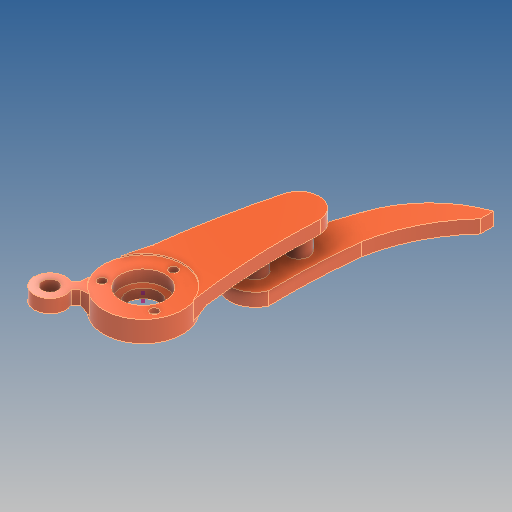
# Autodesk Inventor part: 01-03-01 Zange links nue
Saved by Autodesk Inventor 2026.2 (Build 302298000, 298)
## iProperties
Created: 2025-12-11
Part Number: 01-03-01 Zange links nue
Material: Phenolharz
Document SubType Name: Modeling
Designer: Schally
Density: 1.38 g/cm^3
Appearance: Glatt - Hellorange
Author: Schally
Autodesk Inventor part; units mm, degrees
sketch "Skizze10" plane through (0, 0, 0) normal (1, 0, 0) x (0, 1, 0)
  line L0 (-1.4, 0) -> (8.4, 0) projected
  line L1 (0, -13.2) -> (0, 2.2) projected
  line L2 (2, -2.5) -> (7, -2.5)
  line L3 (7, -2.5) -> (7, -8.5)
  line L4 (7, -8.5) -> (2, -8.5)
  line L5 (2, -8.5) -> (2, -2.5)
  point P0 (0, 0)
  point P1 (0, -11)
  dimension "d135" = 8.5
  dimension "d137" = 5
  dimension "d138" = 2
  dimension "d145" = 2.5
  constraints: 8 end point, 2 parallel, 1 horizontal, 1 perpendicular, 1 point on line
  measures "d135" distance between parallel lines of L0 L4
  measures "d137" distance between parallel lines of L5 L3
  measures "d138" distance between parallel lines of L1 L5
  measures "d145" distance between parallel lines of L0 L2
revolve "Umdrehung2" add sketch "Skizze10" angle 360 about axis through (0, -10, 0) along (0, 1, 0)
ref_plane "Arbeitsebene2" through (0, 6, 0) normal (0, 1, 0) x (1, 0, 0)
ref_plane "Arbeitsebene3" through (0, 4.5, 0) normal (0, 1, 0) x (1, 0, 0)
sketch "Skizze12" plane through (0, 4.5, 0) normal (0, 1, 0) x (1, 0, 0)
  arc A0 (3.5, 80) -> (-11.5, 15.25) centre (296.2619, -21.9337) ccw projected
  arc A1 (28, 100) -> (13, 70) centre (72.0267, 59.2367) ccw projected
  line L0 (28, 100) -> (28, 105) projected
  arc A2 (28, 105) -> (3.5, 80) centre (41.4387, 67.3251) ccw projected
  circle A3 centre (0, 0) radius 15
  arc A4 (13, 70) -> (15, 0) centre (261.1443, 42.0613) ccw
  arc A5 (-11.5, 15.25) -> (-15, 0) centre (120.624, -23.1002) ccw
  circle A6 centre (0, 0) radius 8.5 projected
  line L1 (0, 0) -> (-17.6777, -17.6777)
  line L2 (-87.6656, 0) -> (360.2498, 0) projected
  line L3 (0, 134.1222) -> (0, -49.9776) projected
  circle A7 centre (-17.6777, -17.6777) radius 6
  circle A8 centre (-17.6777, -17.6777) radius 3
  line L4 (1.4142, -1.4142) -> (-12.7279, -15.5563)
  line L5 (-1.4142, 1.4142) -> (-15.5563, -12.7279)
  point P0 (-16.4, 0)
  point P1 (-11.9261, -9.0977)
  point P2 (-15.0919, -12.2635)
  point P3 (-12.2635, -15.0919)
  point P4 (-9.0977, -11.9261)
  dimension "d147" = 30
  dimension "d148" = 45
  dimension "d149" = 25
  dimension "d150" = 12
  dimension "d152" = 3
  dimension "d153" = 2
  dimension "d154" = 2
  constraints: 6 end point, 6 point on circle, 5 centre point, 3 coincident, 2 parallel
  measures "d147" diameter of A3
  measures "d148" angle of L1 L3
  measures "d149" distance of L1.start L1.end
  measures "d150" diameter of A7
  measures "d152" radial gap between concentric circles of A7 A8
  measures "d153" distance between parallel lines of L1 L4
  measures "d154" distance between parallel lines of L1 L5
sketch "Skizze13" plane through (0, 4.5, 0) normal (0, 1, 0) x (1, 0, 0)
  point P0 (0, 0)
extrude "Extrusion8" add sketch "Skizze12" along normal mid plane 5 contours A2 L0 A1 A4 A3 L3 A0 | L3 A3 A5 A0 | L3 A6 L2 A5 A3 | A3 A4 L2 A6 L3 | L3 L2 A6 | A6 L2 L3 | L2 A6 L5 A3 | A3 L3 A6 L2 | A6 L3 L2 | L2 L5 A6 | L3 L4 A6 L1 | L1 A6 L5 L2 | L5 A6 L1 A3 | A3 L1 A7 L5 | A3 L4 A6 L3 | A6 L4 L3 | A6 L4 A3 L1 | A3 L4 A7 L1 | A7
sketch "Skizze14" plane through (0, 4.5, 0) normal (0, 1, 0) x (1, 0, 0)
  circle A0 centre (0, 0) radius 2.5
  dimension "d157" = 5
  constraints: 1 centre point, 1 coincident
  measures "d157" diameter of A0
extrude "Extrusion9" cut sketch "Skizze14" along normal mid plane 20
sketch "Skizze15" plane through (0, 4.5, 0) normal (0, 1, 0) x (1, 0, 0)
  arc A0 (-11.5, 15.25) -> (-15, 0) centre (120.624, -23.1002) ccw projected
  circle A1 centre (0, 0) radius 15
  constraints: 1 coincident, 1 horizontal alignment, 2 other
extrude "Extrusion10" add sketch "Skizze15" along normal mid plane 12
sketch "Skizze16" plane through (0, 4.5, 0) normal (0, 1, 0) x (1, 0, 0)
  circle A0 centre (0, 0) radius 6
  dimension "d162" = 12
  constraints: 1 centre point, 1 coincident
  measures "d162" diameter of A0
extrude "Extrusion11" cut sketch "Skizze16" along normal mid plane 12
sketch "Skizze17" plane through (0, 4.5, 0) normal (0, 1, 0) x (1, 0, 0)
  circle A0 centre (0, 0) radius 8.5
  dimension "d165" = 17
  constraints: 1 centre point, 1 coincident
  measures "d165" diameter of A0
extrude "Extrusion12" cut sketch "Skizze17" along normal mid plane 5
chamfer "Fasen7" distance 2 angle 45 8 edges at (-10.6066, 7, 10.6066) (-9.0977, 5.75, 11.9261) (-9.0977, 3.25, 11.9261) (-10.6066, 2, 10.6066) (0.4428, 2, -14.9935) (0.4428, 7, -14.9935) (-11.9261, 5.75, 9.0977) (-11.9261, 3.25, 9.0977)
sketch "Skizze18" plane through (28, 2, -105) normal (0, -1, 0) x (1, 0, 0)
  point P0 (-28, 105)
ref_plane "Arbeitsebene4" through (28, -7, -105) normal (0, -1, 0) x (1, 0, 0)
sketch "Skizze20" plane through (28, 2, -105) normal (0, -1, 0) x (1, 0, 0)
  circle A0 centre (-24, 50) radius 4
  circle A1 centre (-25.5, 65) radius 4
  point P0 (-28, 105)
  dimension "d188" = 8
  dimension "d189" = 8
  dimension "d192" = 1.5
  dimension "d193" = 15
  constraints: 2 centre point
  measures "d188" diameter of A0
  measures "d189" diameter of A1
  measures "d192" horizontal distance of A1.centre A0.centre
  measures "d193" vertical distance of A1.centre A0.centre
extrude "Extrusion14" add sketch "Skizze20" along normal blind 9
sketch "Skizze19" plane through (28, -7, -105) normal (0, -1, 0) x (1, 0, 0)
  arc A0 (-24.5, 25) -> (0, 0) centre (13.4387, 37.6749) ccw projected
  arc A1 (-15, 35) -> (0, 5) centre (44.0267, 45.7633) ccw projected
  line L0 (0, 0) -> (0, 5) projected
  line L1 (-15, 35) -> (-24.5, 25)
  arc A2 (-39.5, 89.75) -> (-24.5, 25) centre (268.2619, 126.9337) ccw projected
  arc A3 (-14.5526, 94.5996) -> (-15, 35) centre (233.1443, 62.9387) ccw projected
  line L2 (-27, 80) -> (3, 80) construction
  line L3 (-27, 80) -> (-7, 80) construction
  line L4 (-27, 82.5) -> (-5.7868, 82.5) construction
  circle A4 centre (-27, 80) radius 4 projected
  circle A5 centre (-27, 80) radius 4 projected
  circle A6 centre (-27, 60) radius 2.5 projected
  circle A7 centre (-27, 60) radius 2.5 projected
  circle A8 centre (-25.5, 65) radius 4 projected
  circle A9 centre (-25.5, 65) radius 9.7924
  point P0 (-28, 105)
  point P1 (-16.5679, 62.8977)
  point P2 (-37.8031, 77.6969)
  point P3 (-16.4978, 68.8538)
  point P4 (-35.1713, 63.4649)
  constraints: 8 end point, 3 horizontal, 2 point on circle, 1 centre point, 1 coincident
extrude "Extrusion13" add sketch "Skizze19" along normal blind 5 contours L1 A1 L0 A0 | A2 A9 A3 L1 | A2 A9 A3 | A6 A8 | A8 A6 | A6 A8
sketch "Skizze21" plane through (28, 7, -100) normal (0, 1, 0) x (1, 0, 0)
  circle A0 centre (-24, -45) radius 4 projected
  circle A1 centre (-25.5, -60) radius 4 projected
  circle A2 centre (-27, -75) radius 4 projected
  circle A3 centre (-24, -45) radius 7.7999
  arc A4 (-14.5526, -89.5996) -> (-40.5357, -88.5171) centre (-28, -100) ccw projected
  arc A5 (-15, -30) -> (-14.5526, -89.5996) centre (233.1443, -57.9387) ccw projected
  arc A6 (0, 0) -> (-15, -30) centre (44.0267, -40.7633) ccw projected
  line L0 (0, 0) -> (0, 5) projected
  arc A7 (0, 5) -> (-24.5, -20) centre (13.4387, -32.6749) ccw projected
  arc A8 (-24.5, -20) -> (-39.5, -84.75) centre (268.2619, -121.9337) ccw projected
  arc A9 (-39.5, -84.75) -> (-40.5357, -88.5171) centre (92.624, -123.1002) ccw projected
  point P0 (-31.3884, -42.5)
  point P1 (-16.2109, -44.5906)
  constraints: 1 centre point, 1 coincident
extrude "Extrusion15" cut sketch "Skizze21" against normal blind 5 contours A3 A8 A7 L0 A6 A5
sketch "Skizze22" plane through (0, 10.5, 0) normal (0, 1, 0) x (1, 0, 0)
  circle A0 centre (0, 0) radius 15
  constraints: 1 centre point, 1 coincident
extrude "Extrusion16" cut sketch "Skizze22" against normal blind 4
sketch "Skizze23" plane through (0, 6.5, 0) normal (0, 1, 0) x (1, 0, 0)
  circle A0 centre (0, 0) radius 11.5
  circle A1 centre (0, 0) radius 8.5 projected
  arc A2 (-7.4302, -13.0304) -> (14.2414, 4.7098) centre (0, 0) ccw projected
  arc A3 (14.2414, 4.7098) -> (-13.9387, 5.5419) centre (0, 0) ccw projected
  arc A4 (-13.9387, 5.5419) -> (-13.0304, -7.4302) centre (0, 0) ccw projected
  arc A5 (-13.0304, -7.4302) -> (-7.4302, -13.0304) centre (0, 0) ccw projected
  line L0 (0, 0) -> (0, 30.1183)
  line L1 (0, 0) -> (-26.0832, -15.0591)
  line L2 (0, 0) -> (26.0832, -15.0591)
  circle A6 centre (-9.9593, -5.75) radius 1.6
  circle A7 centre (9.9593, -5.75) radius 1.6
  circle A8 centre (0, 11.5) radius 1.6
  dimension "d198" = 3
  dimension "d201" = 360
  dimension "d203" = 3.2
  dimension "d204" = 3.2
  dimension "d205" = 3.2
  dimension "d210" = 23
  constraints: 6 end point, 4 centre point, 3 point on circle, 3 point on line, 1 coincident, 1 vertical, 10 other
  measures "d198" radial gap between concentric circles of A0 A1
  measures "d203" diameter of A6
  measures "d204" diameter of A7
  measures "d205" diameter of A8
  measures "d210" diameter of A0
extrude "Extrusion17" cut sketch "Skizze23" against normal blind 8 contours A8 L0 A0 | A0 L0 A8 | A7 L2 A0 | A0 L2 A7 | L0 A8 A0 | A0 A8 L0 | L2 A7 A0 | A0 A7 L2 | A6 L1 A0 | A0 L1 A6 | A6 L1 A0 | A0 L1 A6
sketch "Skizze24" plane through (0, 7, 0) normal (0, 1, 0) x (0.9991332, 0, 0.0416272)
  arc A0 (-5.779, 57.3091) -> (-12.1248, 14.7581) centre (296.9181, -9.5822) ccw projected
  arc A1 (-12.1248, 14.7581) -> (-13.0028, 10.9511) centre (121.481, -18.0589) ccw projected
  arc A2 (13.0028, 10.9511) -> (-13.0028, 10.9511) centre (0, 0) ccw projected
  arc A3 (9.4724, 55.8521) -> (13.0028, 10.9511) centre (259.167, 52.8955) ccw projected
  line L0 (41.2501, 29.7308) -> (-28.4254, 29.7308)
  line L1 (-28.4254, 29.7308) -> (-28.4254, -36.8887)
  line L2 (-28.4254, -36.8887) -> (41.2501, -36.8887)
  line L3 (41.2501, -36.8887) -> (41.2501, 29.7308)
  point P0 (-10.579, 29.7308)
  point P1 (10.5316, 29.7308)
  constraints: 8 end point, 2 parallel, 1 horizontal, 1 perpendicular
extrude "Extrusion18" cut sketch "Skizze24" along normal blind 5 contours A0 A1 A2 A3 L0 L3 L2 L1
sketch "Skizze26" plane through (0, -1.5, 0) normal (0, -1, 0) x (1, 0, 0)
  circle A0 centre (0, -11.5) radius 1.6 projected
  circle A1 centre (9.9593, 5.75) radius 1.6 projected
  circle A2 centre (-9.9593, 5.75) radius 1.6 projected
  circle A3 centre (-9.9593, 5.75) radius 2.1
  circle A4 centre (9.9593, 5.75) radius 2.1
  circle A5 centre (0, -11.5) radius 2.1
  dimension "d213" = 4.2
  dimension "d214" = 4.2
  dimension "d215" = 4.2
  constraints: 3 centre point, 3 coincident
  measures "d213" diameter of A3
  measures "d214" diameter of A4
  measures "d215" diameter of A5
extrude "Extrusion19" cut sketch "Skizze26" against normal blind 6 contours A0 | A1 | A2 | A3 | A4 | A5
